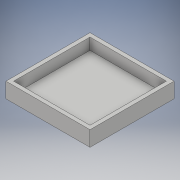
# Autodesk Inventor part: sensor_cover
Saved by Autodesk Inventor 2018 (Build 220112000, 112)
## iProperties
Created: 2018-01-19
Part Number: sensor_cover
Material: Generic
Document SubType Name: Modeling
Designer: matth
Density: 1 g/cm^3
Appearance: Default
Author: matth
Autodesk Inventor part; units mm, degrees
ref_plane "YZ Plane" through (0, 0, 0) normal (1, 0, 0) x (0, 1, 0)
ref_plane "XZ Plane" through (0, 0, 0) normal (0, 1, 0) x (-1, 0, 0)
ref_plane "XY Plane" through (0, 0, 0) normal (0, 0, 1) x (1, 0, 0)
sketch "Sketch1" plane through (0, 0, 0) normal (0, 0, 1) x (1, 0, 0)
  line L0 (-5.3279, 7.3898) -> (14.6721, 7.3898)
  line L1 (14.6721, 7.3898) -> (14.6721, -12.6102)
  line L2 (14.6721, -12.6102) -> (-5.3279, -12.6102)
  line L3 (-5.3279, -12.6102) -> (-5.3279, 7.3898)
  line L4 (-6.3279, 8.3898) -> (15.6721, 8.3898)
  line L5 (15.6721, 8.3898) -> (15.6721, -13.6102)
  line L6 (15.6721, -13.6102) -> (-6.3279, -13.6102)
  line L7 (-6.3279, -13.6102) -> (-6.3279, 8.3898)
  point P0 (0, 0)
  dimension "d0" = 20
  dimension "d1" = 20
  dimension "d2" = 22
  dimension "d3" = 22
  dimension "d4" = 1
  dimension "d5" = 1
  constraints: 16 end point, 4 parallel, 2 horizontal, 2 perpendicular
  measures "d0" distance of L1.end L2.end
  measures "d1" distance of L0.end L1.end
  measures "d2" distance of L5.end L6.end
  measures "d3" distance of L4.end L5.end
  measures "d4" distance between parallel lines of L7 L3
  measures "d5" distance between parallel lines of L4 L0
extrude "Extrusion1" add sketch "Sketch1" along normal blind 3
sketch "Sketch2" plane through (0, 0, 3) normal (0, 0, 1) x (1, 0, 0)
  line L0 (15.6721, 8.3898) -> (-6.3279, 8.3898) projected
  line L1 (-6.3279, -13.6102) -> (15.6721, -13.6102)
  line L2 (15.6721, -13.6102) -> (15.6721, 8.3898)
  line L3 (15.6721, 8.3898) -> (-6.3279, 8.3898)
  line L4 (-6.3279, 8.3898) -> (-6.3279, -13.6102)
  point P0 (0, 0)
  constraints: 8 end point, 2 parallel, 1 horizontal, 1 perpendicular
extrude "Extrusion2" add sketch "Sketch2" along normal blind 1
body "Solid1"
